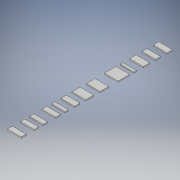
# Autodesk Inventor part: 1st floor interior wall print out.pdf
Saved by Autodesk Inventor 2017 (Build 210142000, 142)
## iProperties
Created: 2018-09-30
Part Number: 1st floor interior wall print out.pdf
Material: Generic
Document SubType Name: Modeling
Designer: User
Density: 1 g/cm^3
Appearance: Default
Author: User
Autodesk Inventor part; units mm, degrees
ref_plane "YZ Plane" through (0, 0, 0) normal (1, 0, 0) x (0, 1, 0)
ref_plane "XZ Plane" through (0, 0, 0) normal (0, 1, 0) x (-1, 0, 0)
ref_plane "XY Plane" through (0, 0, 0) normal (0, 0, 1) x (1, 0, 0)
sketch "Sketch1" plane through (0, 0, 0) normal (0, 1, 0) x (-1, 0, 0)
  line L0 (0, 5.628) -> (63.5, 5.628)
  line L1 (63.5, 5.628) -> (63.5, -17.232)
  line L2 (63.5, -17.232) -> (0, -17.232)
  line L3 (0, -17.232) -> (0, 5.628)
  line L4 (0, -54.7021) -> (63.5, -54.7021)
  line L5 (63.5, -54.7021) -> (63.5, -75.0221)
  line L6 (63.5, -75.0221) -> (0, -75.0221)
  line L7 (0, -75.0221) -> (0, -54.7021)
  line L8 (0, -96.252) -> (63.5, -96.252)
  line L9 (63.5, -96.252) -> (63.5, -116.572)
  line L10 (63.5, -116.572) -> (0, -116.572)
  line L11 (0, -116.572) -> (0, -96.252)
  line L12 (0, -153.8979) -> (63.5, -153.8979)
  line L13 (63.5, -153.8979) -> (63.5, -176.7579)
  line L14 (63.5, -176.7579) -> (0, -176.7579)
  line L15 (0, -176.7579) -> (0, -153.8979)
  line L16 (0, -198.0681) -> (63.5, -198.0681)
  line L17 (63.5, -198.0681) -> (63.5, -213.3081)
  line L18 (63.5, -213.3081) -> (0, -213.3081)
  line L19 (0, -213.3081) -> (0, -198.0681)
  line L20 (0, -241.4897) -> (63.5, -241.4897)
  line L21 (63.5, -241.4897) -> (63.5, -266.8897)
  line L22 (63.5, -266.8897) -> (0, -266.8897)
  line L23 (0, -266.8897) -> (0, -241.4897)
  line L24 (0, -293.1463) -> (63.5, -293.1463)
  line L25 (63.5, -293.1463) -> (63.5, -331.2463)
  line L26 (63.5, -331.2463) -> (0, -331.2463)
  line L27 (0, -331.2463) -> (0, -293.1463)
  line L28 (0, -359.776) -> (63.5, -359.776)
  line L29 (63.5, -359.776) -> (63.5, -400.416)
  line L30 (63.5, -400.416) -> (0, -400.416)
  line L31 (0, -400.416) -> (0, -359.776)
  line L32 (0, -443.9988) -> (63.5, -443.9988)
  line L33 (63.5, -443.9988) -> (63.5, -497.3388)
  line L34 (63.5, -497.3388) -> (0, -497.3388)
  line L35 (0, -497.3388) -> (0, -443.9988)
  line L36 (0, -516.2433) -> (63.5, -516.2433)
  line L37 (63.5, -516.2433) -> (63.5, -528.9433)
  line L38 (63.5, -528.9433) -> (0, -528.9433)
  line L39 (0, -528.9433) -> (0, -516.2433)
  line L40 (0, -560.4135) -> (63.5, -560.4135)
  line L41 (63.5, -560.4135) -> (63.5, -590.8935)
  line L42 (63.5, -590.8935) -> (0, -590.8935)
  line L43 (0, -590.8935) -> (0, -560.4135)
  line L44 (0, -618.0593) -> (63.5, -618.0593)
  line L45 (63.5, -618.0593) -> (63.5, -640.9193)
  line L46 (63.5, -640.9193) -> (0, -640.9193)
  line L47 (0, -640.9193) -> (0, -618.0593)
  line L48 (0, -670.4647) -> (63.5, -670.4647)
  line L49 (63.5, -670.4647) -> (63.5, -695.8647)
  line L50 (63.5, -695.8647) -> (0, -695.8647)
  line L51 (0, -695.8647) -> (0, -670.4647)
  point P0 (0, 0)
  dimension "d0" = 63.5
  dimension "d1" = 22.86
  dimension "d2" = 20.32
  dimension "d3" = 20.32
  dimension "d4" = 63.5
  dimension "d5" = 22.86
  dimension "d6" = 15.24
  dimension "d7" = 63.5
  dimension "d8" = 25.4
  dimension "d9" = 63.5
  dimension "d10" = 38.1
  dimension "d11" = 63.5
  dimension "d12" = 40.64
  dimension "d13" = 63.5
  dimension "d14" = 53.34
  dimension "d15" = 12.7
  dimension "d16" = 30.48
  dimension "d17" = 22.86
  dimension "d18" = 63.5
  dimension "d19" = 25.4
  constraints: 104 end point, 40 point on line, 35 perpendicular, 3 horizontal
  measures "d0" distance of L0.start L0.end
  measures "d1" distance of L0.end L1.end
  measures "d2" distance of L4.end L5.end
  measures "d3" distance of L8.end L9.end
  measures "d4" distance of L12.start L12.end
  measures "d5" distance of L12.end L13.end
  measures "d6" distance of L16.end L17.end
  measures "d7" distance of L20.start L20.end
  measures "d8" distance of L20.end L21.end
  measures "d9" distance of L24.start L24.end
  measures "d10" distance of L24.end L25.end
  measures "d11" distance of L28.start L28.end
  measures "d12" distance of L28.end L29.end
  measures "d13" distance of L32.start L32.end
  measures "d14" distance of L32.end L33.end
  measures "d15" distance of L36.end L37.end
  measures "d16" distance of L40.end L41.end
  measures "d17" distance of L44.end L45.end
  measures "d18" distance of L48.start L48.end
  measures "d19" distance of L48.end L49.end
extrude "Extrusion1" add sketch "Sketch1" along normal blind 5.08
body "Solid1"
